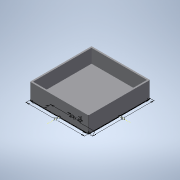
# Autodesk Inventor part: Enclosure
Saved by Autodesk Inventor 2022 (Build 260153000, 153)
## iProperties
Created: 2023-10-31
Part Number: Enclosure
Material: Generic
Document SubType Name: Modeling
Designer: Baaij
Density: 1 g/cm^3
Appearance: Default
Author: Baaij
Autodesk Inventor part; units mm, degrees
ref_plane "YZ Plane" through (0, 0, 0) normal (1, 0, 0) x (0, 1, 0)
ref_plane "XZ Plane" through (0, 0, 0) normal (0, 1, 0) x (-1, 0, 0)
ref_plane "XY Plane" through (0, 0, 0) normal (0, 0, 1) x (1, 0, 0)
sketch "Sketch_BoxBase" plane through (0, 0, 0) normal (0, 0, 1) x (1, 0, 0)
  line L0 (0, 56.7) -> (0, -56.7) construction
  line L1 (-53.9, 0) -> (53.9, 0) construction
  line L2 (-36.5, 38.5) -> (36.5, 38.5)
  line L3 (36.5, 38.5) -> (36.5, -38.5)
  line L4 (36.5, -38.5) -> (-36.5, -38.5)
  line L5 (-36.5, -38.5) -> (-36.5, 38.5)
  line L6 (-36.5, 38.5) -> (36.5, -38.5) construction
  line L7 (36.5, 38.5) -> (-36.5, -38.5) construction
  line L8 (-38.5, 40.5) -> (38.5, 40.5)
  line L9 (38.5, 40.5) -> (38.5, -40.5)
  line L10 (38.5, -40.5) -> (-38.5, -40.5)
  line L11 (-38.5, -40.5) -> (-38.5, 40.5)
  line L12 (-38.5, 40.5) -> (38.5, -40.5) construction
  line L13 (38.5, 40.5) -> (-38.5, -40.5) construction
  point P0 (0, 0)
  point P1 (-20, -33.5)
  point P2 (20, -33.5)
  dimension "d4" = 73
  dimension "d5" = 77
  dimension "d6" = 77
  dimension "d7" = 81
  dimension "d23" = 40
  dimension "d24" = 20
  dimension "d25" = 7
  dimension "d26" = 7
  constraints: 24 end point, 4 midpoint, 4 parallel, 2 horizontal, 2 perpendicular
  measures "d4" distance of L3.end L4.end
  measures "d5" distance of L2.end L3.end
  measures "d6" distance of L9.end L10.end
  measures "d7" distance of L8.end L9.end
  measures "d23" distance of point (20, -33.5) point (-20, -33.5)
  measures "d24" distance from line of L0 point (20, -33.5)
  measures "d25" distance from line of L10 point (-20, -33.5)
  measures "d26" distance from line of L10 point (20, -33.5)
extrude "Extr_Edge" add sketch "Sketch_BoxBase" along normal blind 21
extrude "Extr_Bottom" add sketch "Sketch_BoxBase" along normal blind 3 contours L2 L3 L4 L5
hole "Hole2" at (-20, -33.5, 0) at (20, -33.5, 0) direction (0, 0, 1) diameter 4 end through all
fillet "Fillet1" radius 1 1 edges at (38.5, 40.5, 10.5)
fillet "Fillet2" radius 1 4 edges at (-38.5, 40.5, 10.5) (-38.5, -40.5, 10.5) (38.5, -40.5, 10.5) (-38.5, 0, 0)
equation "\"d24\" = 0.5 * d23"
equation "\"d26\" = d25"
body "Solid3"
